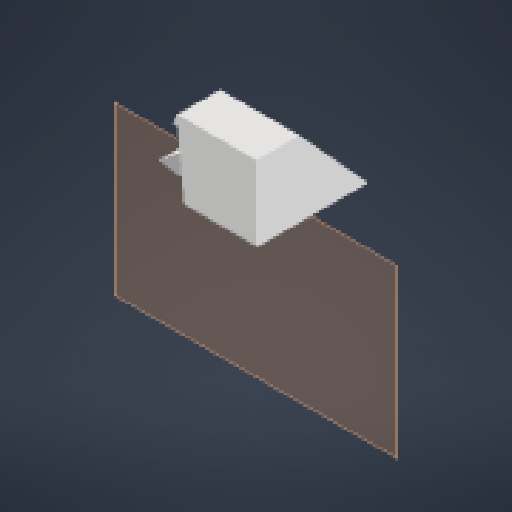
# Autodesk Inventor part: Head_Fin
Saved by Autodesk Inventor 2024 (Build 280153000, 153)
## iProperties
Created: 2025-09-25
Part Number: Head_Fin
Material: Generic
Document SubType Name: Modeling
Designer: kevin
Density: 1 g/cm^3
Appearance: Default
Author: kevin
Autodesk Inventor part; units mm, degrees
ref_plane "YZ Plane" through (0, 0, 0) normal (1, 0, 0) x (0, 1, 0)
ref_plane "XZ Plane" through (0, 0, 0) normal (0, 1, 0) x (-1, 0, 0)
ref_plane "XY Plane" through (0, 0, 0) normal (0, 0, 1) x (1, 0, 0)
ref_plane "Work Plane1" through (0, 0, 0) normal (0, 0, 1) x (1, 0, 0)
sketch "Sketch1" plane through (0, 0, 0) normal (0, 0, 1) x (1, 0, 0)
  line L0 (-38.0834, 109.3576) -> (68.9757, 109.3576) projected
  line L1 (-38.0834, 138.5676) -> (68.9757, 138.5676)
  line L2 (68.4541, 109.3576) -> (43.944, 138.5676)
  line L3 (68.4541, 109.3576) -> (106.585, 109.3576) construction
  line L4 (-18.3608, 138.5676) -> (-18.3608, 134.5676)
  line L5 (-18.3608, 134.5676) -> (-14.3608, 134.5676)
  line L6 (-14.3608, 134.5676) -> (10.8492, 109.3576)
  point P0 (0, 0)
  dimension "d0" = 29.21
  dimension "d1" = 130
  dimension "d2" = 4
  dimension "d3" = 4
  constraints: 12 end point, 4 point on line, 2 perpendicular, 1 equal length, 1 horizontal, 1 parallel
  measures "d0" distance between parallel lines of L0 L1
  measures "d1" angle of L3 L2
  measures "d2" distance of L4.start L4.end
  measures "d3" distance of L4.end L5.end
extrude "Extrusion1" add sketch "Sketch1" along normal mid plane 78.6511
sketch "Sketch2" plane through (0, 0, 0) normal (0, 0, 1) x (1, 0, 0)
  line L0 (-38.0834, 109.3576) -> (68.9757, 109.3576) projected
  line L1 (10.8492, 109.3576) -> (-14.3608, 134.5676) projected
  line L2 (-5.5484, 125.7552) -> (-25.9454, 109.3576)
  point P0 (0, 0)
  constraints: 2 end point, 2 point on line
extrude "Extrusion2" add sketch "Sketch2" along normal mid plane 45.7835
chamfer "Chamfer1" distance 28.575 angle 40 1 edges at (12.7916, 138.5676, -39.3255) measured on face at (41.0824, 119.0943, -39.3256)
chamfer "Chamfer2" distance 28.575 angle 40 1 edges at (12.7916, 138.5676, 39.3255) measured on face at (41.0824, 119.0943, 39.3256)
chamfer "Chamfer3" distance 7.9375 angle 15 1 edges at (-15.7469, 117.5564, -22.8918) measured on face at (-6.8815, 114.8235, -22.8918)
chamfer "Chamfer4" distance 7.9375 angle 15 1 edges at (-15.7469, 117.5564, 22.8918) measured on face at (-6.8815, 114.8235, 22.8918)
sketch "Sketch3" plane through (10.8492, 109.3576, -39.3255) normal (0, -1, 0) x (1, 0, 0)
  circle A0 centre (18.7843, 31.3255) radius 2.1 projected
  circle A1 centre (-6.2157, 31.3255) radius 2.1 projected
  circle A2 centre (-6.2157, 47.3255) radius 2.1 projected
  circle A3 centre (18.7843, 47.3255) radius 2.1 projected
  point P0 (-10.8492, 39.3255)
extrude "Extrusion3" cut sketch "Sketch3" against normal blind 15
body "Solid1"
